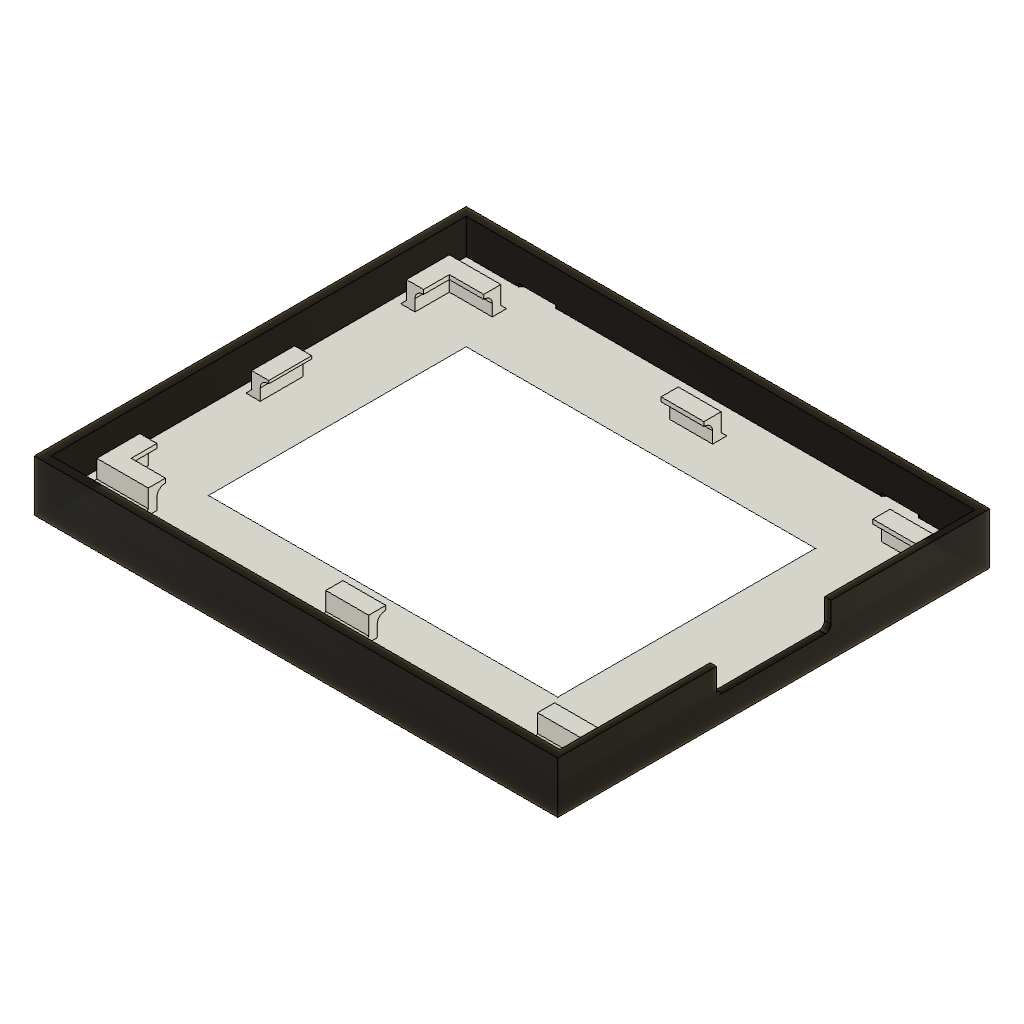
paperwhite_3 (Autodesk Fusion 360 design; units mm, degrees)
Autodesk Fusion 360 part; units mm, degrees
note: some values were not read from the file. Chosen so that the rebuilt part matches the saved one: which face or edge a step refers to; which pieces of a blend or face edit are solid. Set by a fixed rule: which sketch regions a step uses.
sketch "Sketch1" plane through (0, 0, 0) normal (0, 0, 1) x (1, 0, 0)
  line L0 (0, 0) -> (122, 0)
  line L1 (122, 0) -> (122, -90)
  line L2 (122, -90) -> (0, -90)
  line L3 (0, -90) -> (0, 0)
  line L4 (149.5, -117.5) -> (-27.5, -117.5)
  line L5 (-27.5, -117.5) -> (-27.5, 27.5)
  line L6 (-27.5, 27.5) -> (149.5, 27.5)
  line L7 (149.5, 27.5) -> (149.5, -117.5)
  line L8 (122, -45) -> (0, -45) construction
  line L9 (61, -45) -> (61, 0) construction
  line L10 (61, -45) -> (65, -45) construction
  line L11 (149.5, 13.6) -> (-19.5, 13.6)
  line L12 (-19.5, 13.6) -> (-19.5, -103.6)
  line L13 (-19.5, -103.6) -> (149.5, -103.6)
  line L14 (149.5, -103.6) -> (149.5, 13.6)
  line L15 (149.5, 13.6) -> (-19.5, -103.6) construction
  line L16 (-19.5, 13.6) -> (149.5, -103.6) construction
  line L17 (146.5, 13.6) -> (131.5, 13.6)
  line L18 (131.5, 13.6) -> (131.5, 16.6)
  line L19 (131.5, 16.6) -> (146.5, 16.6)
  line L20 (146.5, 16.6) -> (146.5, 13.6)
  line L21 (-24.5, 24.5) -> (146.5, 24.5)
  line L22 (146.5, 24.5) -> (146.5, -114.5)
  line L23 (146.5, -114.5) -> (-24.5, -114.5)
  line L24 (-24.5, -114.5) -> (-24.5, 24.5)
  line L25 (152.5, 30.5) -> (152.5, -120.5)
  line L26 (152.5, -120.5) -> (-30.5, -120.5)
  line L27 (-30.5, -120.5) -> (-30.5, 30.5)
  line L28 (-30.5, 30.5) -> (152.5, 30.5)
  line L29 (72.5, 13.6) -> (57.5, 13.6)
  line L30 (57.5, 13.6) -> (57.5, 16.6)
  line L31 (57.5, 16.6) -> (72.5, 16.6)
  line L32 (72.5, 16.6) -> (72.5, 13.6)
  line L33 (-19.5, 13.6) -> (-4.5, 13.6)
  line L34 (-4.5, 13.6) -> (-4.5, 16.6)
  line L35 (-4.5, 16.6) -> (-22.5, 16.6)
  line L36 (-19.5, -37.5) -> (-22.5, -37.5)
  line L37 (-22.5, -37.5) -> (-22.5, -52.5)
  line L38 (-22.5, -52.5) -> (-19.5, -52.5)
  line L39 (-19.5, -52.5) -> (-19.5, -37.5)
  line L40 (146.5, -103.6) -> (131.5, -103.6)
  line L41 (131.5, -103.6) -> (131.5, -106.6)
  line L42 (131.5, -106.6) -> (146.5, -106.6)
  line L43 (146.5, -106.6) -> (146.5, -103.6)
  line L44 (72.5, -103.6) -> (57.5, -103.6)
  line L45 (57.5, -103.6) -> (57.5, -106.6)
  line L46 (57.5, -106.6) -> (72.5, -106.6)
  line L47 (72.5, -106.6) -> (72.5, -103.6)
  line L48 (-4.5, -103.6) -> (-19.5, -103.6)
  line L49 (-19.5, -106.6) -> (-4.5, -106.6)
  line L50 (-4.5, -106.6) -> (-4.5, -103.6)
  line L51 (-19.5, -106.6) -> (-22.5, -106.6)
  line L52 (-22.5, -106.6) -> (-22.5, -91.6)
  line L53 (-22.5, -91.6) -> (-19.5, -91.6)
  line L54 (-19.5, -91.6) -> (-19.5, -103.6)
  line L55 (-22.5, 16.6) -> (-22.5, 1.6)
  line L56 (-22.5, 1.6) -> (-19.5, 1.6)
  line L57 (-19.5, 1.6) -> (-19.5, 13.6)
  line L58 (146.5, -103.6) -> (131.5, -103.6)
  line L59 (131.5, -103.6) -> (131.5, -100.6)
  line L60 (131.5, -100.6) -> (146.5, -100.6)
  line L61 (146.5, -100.6) -> (146.5, -103.6)
  line L62 (72.5, -103.6) -> (57.5, -103.6)
  line L63 (57.5, -103.6) -> (57.5, -100.6)
  line L64 (57.5, -100.6) -> (72.5, -100.6)
  line L65 (72.5, -100.6) -> (72.5, -103.6)
  line L66 (-4.5, -103.6) -> (-19.5, -103.6)
  line L67 (-16.5, -100.6) -> (-4.5, -100.6)
  line L68 (-4.5, -100.6) -> (-4.5, -103.6)
  line L69 (-19.5, -52.5) -> (-16.5, -52.5)
  line L70 (-16.5, -52.5) -> (-16.5, -37.5)
  line L71 (-16.5, -37.5) -> (-19.5, -37.5)
  line L72 (-19.5, -37.5) -> (-19.5, -52.5)
  line L73 (-19.5, -91.6) -> (-16.5, -91.6)
  line L74 (-16.5, -91.6) -> (-16.5, -100.6)
  line L75 (-4.5, 13.6) -> (-19.5, 13.6)
  line L76 (-16.5, 10.6) -> (-4.5, 10.6)
  line L77 (-4.5, 10.6) -> (-4.5, 13.6)
  line L78 (-19.5, 1.6) -> (-16.5, 1.6)
  line L79 (-19.5, 11) -> (-19.5, 1.6)
  line L80 (131.5, 16.6) -> (131.5, 10.6)
  line L81 (131.5, 10.6) -> (146.5, 10.6)
  line L82 (146.5, 10.6) -> (146.5, 13.6)
  line L83 (72.5, 13.6) -> (57.5, 13.6)
  line L84 (57.5, 13.6) -> (57.5, 10.6)
  line L85 (57.5, 10.6) -> (72.5, 10.6)
  line L86 (72.5, 10.6) -> (72.5, 13.6)
  line L87 (-16.5, 1.6) -> (-16.5, 10.6)
  point P0 (65, -45)
  dimension "d15" = 122
  dimension "d16" = 90
  dimension "d18" = 4
  dimension "d19" = 169
  dimension "d20" = 117.2
  dimension "d21" = 15
  dimension "d22" = 3
  dimension "d25" = 3
  dimension "d40" = 15
  dimension "d41" = 15
  dimension "d43" = 3
  dimension "d45" = 3
  dimension "d46" = 15
  dimension "d59" = 15
  dimension "d61" = 15
  dimension "d63" = 3
  dimension "d64" = 3
  dimension "d68" = 3
  dimension "d72" = 15
  dimension "d73" = 3
  dimension "d126" = 27.5
  dimension "d127" = 27.5
  dimension "d129" = 27.5
  dimension "d130" = 27.5
  constraint horizontal L0
  constraint vertical L1
  constraint horizontal L2
  constraint vertical L3
  constraint coincident L0.start L3.end
  constraint midpoint L1 L8.start
  constraint midpoint L3 L8.end
  constraint midpoint L8 L9.start
  constraint midpoint L0 L9.end
  constraint perpendicular L9 L10
  constraint horizontal L11
  constraint perpendicular L11 L12
  constraint parallel L11 L13
  constraint parallel L12 L14
  constraint coincident L15 P0
  constraint coincident L16 P0
  constraint coincident P0 L10.end
  constraint horizontal L17
  constraint vertical L18
  constraint horizontal L19
  constraint vertical L20
  constraint coincident L11 L17.start
  constraint horizontal L29
  constraint vertical L30
  constraint horizontal L31
  constraint vertical L32
  constraint coincident L11 L29.start
  constraint horizontal L33
  constraint vertical L34
  constraint horizontal L35
  constraint horizontal L36
  constraint vertical L37
  constraint horizontal L38
  constraint vertical L39
  constraint coincident L12 L36.start
  constraint horizontal L40
  constraint vertical L41
  constraint horizontal L42
  constraint vertical L43
  constraint coincident L13 L40.start
  constraint coincident L22 L40.start
  constraint horizontal L44
  constraint vertical L45
  constraint horizontal L46
  constraint vertical L47
  constraint coincident L13 L44.start
  constraint horizontal L48
  constraint horizontal L49
  constraint vertical L50
  constraint coincident L13 L48.start
  constraint horizontal L51
  constraint vertical L52
  constraint horizontal L53
  constraint vertical L54
  constraint vertical L55
  constraint horizontal L56
  constraint vertical L57
  constraint horizontal L58
  constraint vertical L59
  constraint horizontal L60
  constraint vertical L61
  constraint horizontal L62
  constraint vertical L63
  constraint horizontal L64
  constraint vertical L65
  constraint horizontal L66
  constraint horizontal L67
  constraint vertical L68
  constraint horizontal L69
  constraint vertical L70
  constraint horizontal L71
  constraint vertical L72
  constraint horizontal L73
  constraint vertical L74
  constraint horizontal L75
  constraint horizontal L76
  constraint vertical L77
  constraint horizontal L78
  constraint vertical L87
  constraint vertical L79
  constraint vertical L80
  constraint horizontal L81
  constraint vertical L82
  constraint horizontal L83
  constraint vertical L84
  constraint horizontal L85
  constraint vertical L86
  constraint coincident L20 L17.start
  constraint midpoint L13 L62
  constraint midpoint L11 L29
  constraint equal L53 L73
  constraint coincident L12 L13.start
  constraint midpoint L12 L72
  constraint equal L37 L70
  constraint equal L36 L71
  constraint equal L31 L85
  constraint equal L42 L60
  constraint equal L41 L59
  constraint equal L32 L86
  constraint equal L46 L64
  constraint equal L47 L65
  constraint equal L49 L52
  constraint equal L50 L68
  constraint equal L68 L73
  constraint equal L48 L52
  constraint equal L20 L82
  constraint equal L19 L81
  constraint coincident L19 L18.end
  constraint coincident L22 L17.start
  constraint equal L34 L77
  constraint coincident L11.end L12.start
  constraint equal L77 L78
  constraint equal L56 L78
  constraint equal L55 L75
  constraint coincident L11.end L12
  measures "d15" distance of L0.start L0.end
  measures "d16" distance of L0.start L2.end
  measures "d18" distance of L9.start P0
  measures "d19" distance of L12.end L13.end
  measures "d20" distance of L11.end L12.end
  measures "d21" distance of L17.start L17.end
  measures "d22" distance of L17.start L19.end
  measures "d40" distance of L11.end L33.end
  measures "d41" distance of L36.start L38.end
  measures "d43" distance of L40.start L42.end
  measures "d45" distance of L44.start L46.end
  measures "d46" distance of L48.start L12.end
  measures "d59" distance of L40.start L40.end
  measures "d61" distance of L44.start L44.end
  measures "d63" distance of L48.start L67.end
  measures "d64" distance of L38.end L69.end
  measures "d68" distance of L33.end L76.end
  measures "d72" distance of L29.start L29.end
  measures "d73" distance of L29.start L85.end
  measures "d126" distance of L0 L6
  measures "d127" distance of L2 L4
  measures "d129" distance of L1 L7
  measures "d130" distance of L3 L5
extrude "Extrude4" add sketch "Sketch1" along normal blind 1 contours L4 L5 L6 L7 L11 L13 L20 L21 L22 L23 L24 L43 | L7 L11 L13 L14 L22 L61 L82 | L13 L22 L40 L41 L42 L43 L58 | L13 L22 L40 L58 L59 L60 L61 | L11 L17 L22 L80 L81 L82 | L11 L17 L18 L19 L20 L22 L80 | L11 L12 L13 L18 L19 L21 L22 L23 L24 L30 L31 L32 L34 L35 L36 L37 L38 L41 L42 L45 L46 L47 L49 L50 L51 L52 L53 L55 L56 L80 | L11 L12 L13 L22 L59 L60 L63 L64 L65 L67 L68 L69 L70 L71 L73 L74 L76 L77 L78 L80 L81 L84 L85 L86 L87 | L13 L44 L45 L46 L47 L62 | L13 L44 L62 L63 L64 L65 | L11 L29 L83 L84 L85 L86 | L11 L29 L30 L31 L32 L83 | L12 L13 L48 L49 L50 L51 L52 L53 L54 L66 | L12 L13 L48 L54 L66 L67 L68 L73 L74 | L11 L12 L33 L57 L75 L76 L77 L78 L79 L87 | L11 L12 L33 L34 L35 L55 L56 L57 L75 L79 | L12 L36 L37 L38 L39 L72 | L12 L39 L69 L70 L71 L72 makes body 1
sketch "Sketch2" plane through (154.5, 0, 0) normal (1, 0, 0) x (0, 1, 0)
  line L0 (-122.5, 13) -> (-122.5, 0)
  line L1 (32.5, 0) -> (32.5, 13)
  line L2 (32.5, 13) -> (-122.5, 13)
  line L3 (27.5, 1) -> (-117.5, 1)
  line L4 (-45, 0) -> (-45, 13)
  line L5 (-45, 13) -> (-65, 13) construction
  line L6 (-65, 13) -> (-25, 13)
  line L7 (-25, 13) -> (-25, 3.8)
  line L8 (-25, 3.8) -> (-65, 3.8)
  line L9 (-65, 3.8) -> (-65, 13)
  line L10 (-122.5, 0) -> (32.5, 0)
  point P0 (-45, 0)
  dimension "d31" = 20
  dimension "d32" = 40
  dimension "d132" = 9.2
  constraint coincident P0 L4.start
  constraint perpendicular L3 L4
  constraint perpendicular L4 L5
  constraint horizontal L6
  constraint vertical L7
  constraint horizontal L8
  constraint vertical L9
  constraint coincident L2 L5.end
  measures "d31" distance of L4.end L5.end
  measures "d32" distance of L5.end L6.end
  measures "d132" distance of L6 L8
extrude "Extrude7" add sketch "Sketch1" against normal blind 5 separate body contours L4 L5 L6 L7 L11 L13 L20 L21 L22 L23 L24 L43 | L7 L11 L13 L14 L22 L61 L82 | L25 L26 L27 L28 makes body 2
extrude "Extrude8" add sketch "Sketch1" along normal blind 13 contours L25 L26 L27 L28 bodies 2
chamfer "Chamfer1" distance 1 angle 45 4 edges at (122, -45, 0) (61, 0, 0) (0, -45, 0) (61, -90, 0) on bodies 1
extrude "Extrude9" add sketch "Sketch1" along normal blind 7.8 from surface at 1 contours L13 L22 L40 L41 L42 L43 L58 | L11 L17 L18 L19 L20 L22 L80 | L13 L44 L45 L46 L47 L62 | L11 L29 L30 L31 L32 L83 | L12 L13 L48 L49 L50 L51 L52 L53 L54 L66 | L11 L12 L33 L34 L35 L55 L56 L57 L75 L79 | L12 L36 L37 L38 L39 L72 bodies 1
chamfer "Chamfer2" distance 2 angle 45 9 edges at (139, 16.6, 1) (65, 16.6, 1) (-13.5, 16.6, 1) (-22.5, 9.1, 1) (-22.5, -45, 1) (-22.5, -99.1, 1) (-13.5, -106.6, 1) (65, -106.6, 1) (139, -106.6, 1) on bodies 1
extrude "Extrude10" cut sketch "Sketch2" against normal blind 5 contours L2 L4 L6 L8 L9 | L2 L4 L6 L7 L8 bodies 2
fillet "Fillet1" radius 2 2 edges at (151, -65, 3.8) (151, -25, 3.8) on bodies 2
extrude "Extrude11" add sketch "Sketch1" against normal blind 1 from surface at 8.8 contours L13 L22 L40 L58 L59 L60 L61 | L11 L17 L22 L80 L81 L82 | L13 L44 L62 L63 L64 L65 | L11 L29 L83 L84 L85 L86 | L12 L13 L48 L54 L66 L67 L68 L73 L74 | L11 L12 L33 L57 L75 L76 L77 L78 L79 L87 | L12 L39 L69 L70 L71 L72 bodies 1
extrude "Extrude12" add 6 faces at (141.5, -104.6, 8.8) (62.5, -105.6, 8.8) (-20.5, -99.6, 8.8) (-14.5, 14.6, 8.8) (67.5, 13.6, 8.8) (141.5, 12.6, 8.8) along direction (0, 0, 1) blind 0.5 on bodies 1 bodies 1
move_face "OffsetFaces3" offset -0.2 4 faces at (31.5, 27.5, 0.6667) (149.5, -20.8333, 0.6667) (90.5, -117.5, 0.6667) (-27.5, -69.1667, 0.6667) on bodies 1
sketch "Sketch3" plane through (0, -117.5, 0) normal (0, 1, 0) x (-1, 0, 0)
  line L0 (-149.5, 0) -> (27.5, 0)
  line L1 (27.5, 0) -> (27.5, 13)
  line L2 (27.5, 13) -> (-149.5, 13)
  line L3 (-149.5, 13) -> (-149.5, 0)
  line L4 (-125, 1) -> (-62, 1)
  line L5 (-62, 1) -> (-62, -9)
  line L6 (-62, -9) -> (-125, -9)
  line L7 (-125, -9) -> (-125, 1)
  line L8 (27.3, 1) -> (-149.3, 1)
  line L9 (-125, 1) -> (-115, 1)
  line L10 (-115, 1) -> (-115, 3)
  line L11 (-115, 3) -> (-125, 3)
  line L12 (-125, 3) -> (-125, 1)
  dimension "d80" = 10
  dimension "d81" = 2
  constraint horizontal L4
  constraint vertical L5
  constraint horizontal L6
  constraint vertical L7
  constraint coincident L4.start L8
  constraint horizontal L9
  constraint vertical L10
  constraint horizontal L11
  constraint vertical L12
  measures "d80" distance of L4.start L9.end
  measures "d81" distance of L4.start L11.end
fillet "Fillet2" radius 2.75 9 edges at (65, 13.6, 7.8) (139, 13.6, 7.8) (-12, 13.6, 7.8) (-19.5, 7.6, 7.8) (-19.5, -45, 7.8) (-12, -103.6, 7.8) (-19.5, -97.6, 7.8) (65, -103.6, 7.8) (139, -103.6, 7.8) on bodies 1
sketch "Sketch4" plane through (0, 0, 1) normal (0, 0, 1) x (-1, 0, 0)
  line L0 (-149.3, 117.3) -> (-149.3, -27.3)
  line L1 (-149.3, -27.3) -> (27.3, -27.3)
  line L2 (27.3, 117.3) -> (-149.3, 117.3)
  line L3 (-122, 0) -> (-122, 90)
  line L4 (27.5, 45) -> (-149.3, 45) construction
  line L5 (7.5, -27.3) -> (-2.5, -27.3)
  line L6 (-2.5, -27.3) -> (-2.5, -28.8)
  line L7 (-2.5, -28.8) -> (7.5, -28.8)
  line L8 (7.5, -28.8) -> (7.5, -27.3)
  line L9 (-129.3, -27.3) -> (-119.3, -27.3)
  line L10 (-119.3, -27.3) -> (-119.3, -28.8)
  line L11 (-119.3, -28.8) -> (-129.3, -28.8)
  line L12 (-129.3, -28.8) -> (-129.3, -27.3)
  line L13 (7.5, -28.8) -> (9, -27.3)
  line L14 (7.5, -28.8) -> (9.6213, -28.8) construction
  line L15 (-2.5, -28.8) -> (-4, -27.3)
  line L16 (-119.3, -28.8) -> (-117.8, -27.3)
  line L17 (-129.3, -28.8) -> (-130.8, -27.3)
  line L18 (7.5, 118.8) -> (7.5, 117.3)
  line L19 (7.5, 118.8) -> (9, 117.3)
  line L20 (-2.5, 118.8) -> (7.5, 118.8)
  line L21 (7.5, 117.3) -> (-2.5, 117.3)
  line L22 (-2.5, 117.3) -> (-2.5, 118.8)
  line L23 (-2.5, 118.8) -> (-4, 117.3)
  line L24 (-119.3, 118.8) -> (-117.8, 117.3)
  line L25 (-119.3, 117.3) -> (-119.3, 118.8)
  line L26 (-129.3, 117.3) -> (-119.3, 117.3)
  line L27 (-119.3, 118.8) -> (-129.3, 118.8)
  line L28 (-129.3, 118.8) -> (-129.3, 117.3)
  line L29 (-129.3, 118.8) -> (-130.8, 117.3)
  line L30 (27.5, 117.5) -> (27.5, -27.5)
  line L31 (-131.5, 108.6) -> (-131.5, 103.6)
  line L32 (-131.5, 103.6) -> (-146.5, 103.6)
  line L33 (-146.5, 103.6) -> (-146.5, 108.6)
  line L34 (-146.5, 108.6) -> (-131.5, 108.6)
  line L35 (-146.5, -18.6) -> (-146.5, -13.6)
  line L36 (-146.5, -13.6) -> (-131.5, -13.6)
  line L37 (-131.5, -13.6) -> (-131.5, -18.6)
  line L38 (-131.5, -18.6) -> (-146.5, -18.6)
  line L39 (-57.5, 108.6) -> (-57.5, 103.6)
  line L40 (-57.5, 103.6) -> (-72.5, 103.6)
  line L41 (-72.5, 103.6) -> (-72.5, 108.6)
  line L42 (-72.5, 108.6) -> (-57.5, 108.6)
  line L43 (-72.5, -18.6) -> (-72.5, -13.6)
  line L44 (-72.5, -13.6) -> (-57.5, -13.6)
  line L45 (-57.5, -13.6) -> (-57.5, -18.6)
  line L46 (-57.5, -18.6) -> (-72.5, -18.6)
  line L47 (27.3, -27.3) -> (27.3, 117.3)
  line L48 (-122, 90) -> (0, 90)
  line L49 (0, 90) -> (0, 0)
  line L50 (0, 0) -> (-122, 0)
  line L51 (4.5, 103.6) -> (4.5, 108.6)
  line L52 (4.5, 108.6) -> (24.5, 108.6)
  line L53 (24.5, 91.6) -> (19.5, 91.6)
  line L54 (19.5, 91.6) -> (19.5, 103.6)
  line L55 (19.5, 103.6) -> (4.5, 103.6)
  line L56 (19.5, -1.6) -> (24.5, -1.6)
  line L57 (24.5, -18.6) -> (4.5, -18.6)
  line L58 (4.5, -18.6) -> (4.5, -13.6)
  line L59 (4.5, -13.6) -> (19.5, -13.6)
  line L60 (19.5, -13.6) -> (19.5, -1.6)
  line L61 (24.5, 37.5) -> (19.5, 37.5)
  line L62 (19.5, 37.5) -> (19.5, 52.5)
  line L63 (19.5, 52.5) -> (24.5, 52.5)
  line L64 (24.5, 108.6) -> (24.5, 91.6)
  line L65 (24.5, -1.6) -> (24.5, -18.6)
  line L66 (24.5, 52.5) -> (24.5, 37.5)
  dimension "d84" = 10
  dimension "d85" = 1.5
  dimension "d86" = 10
  dimension "d87" = 1.5
  dimension "d88" = 45
  dimension "d121" = 20
  dimension "d122" = 20
  constraint midpoint L0 L4.end
  constraint horizontal L5
  constraint vertical L6
  constraint horizontal L7
  constraint vertical L8
  constraint coincident L1 L5.start
  constraint horizontal L9
  constraint vertical L10
  constraint horizontal L11
  constraint vertical L12
  constraint coincident L1 L9.start
  constraint horizontal L14
  constraint coincident L1 L13.end
  constraint coincident L1 L15.end
  constraint perpendicular L13 L15
  constraint coincident L1 L16.end
  constraint perpendicular L15 L16
  constraint coincident L1 L17.end
  constraint perpendicular L16 L17
  constraint symmetric L4 L5.start L18.end
  constraint symmetric L4 L5.end L21.end
  constraint symmetric L4 L6.end L20.start
  constraint symmetric L4 L7.end L18.start
  constraint symmetric L4 L9.start L26.start
  constraint symmetric L4 L9.end L25.start
  constraint symmetric L4 L10.end L24.start
  constraint symmetric L4 L11.end L27.end
  constraint symmetric L4 L13.end L19.end
  constraint symmetric L4 L15.end L23.end
  constraint symmetric L4 L16.end L24.end
  constraint symmetric L4 L17.end L29.end
  constraint midpoint L4.start L30
  measures "d84" distance of L5.start L5.end
  measures "d85" distance of L5.start L7.end
  measures "d86" distance of L9.start L9.end
  measures "d87" distance of L9.start L11.end
  measures "d88" angle of L13 L14
  measures "d121" distance of L8 L30
  measures "d122" distance of L0 L12
extrude "Extrude13" add 1 faces at (149.3, -20.9, 0.6667) along direction (1, 0, 0) blind 0.75 on bodies 1 bodies 1
extrude "Extrude14" cut 1 faces at (149.5, 10, 6.2667) along direction (1, 0, 0) blind 0.75 on bodies 2 bodies 2
extrude "Extrude15" add sketch "Sketch4" against normal blind 1 contours L2 L28 L29 | L1 L12 L17 | L2 L25 L26 L27 L28 | L1 L9 L10 L11 L12 | L2 L24 L25 | L1 L10 L16 | L2 L22 L23 | L1 L6 L15 | L2 L18 L20 L21 L22 | L1 L5 L6 L7 L8 | L2 L18 L19 | L1 L8 L13 bodies 1
chamfer "Chamfer3" distance 0.3 angle 45 8 edges at (124.3, 28.8, 1) (124.3, 28.8, 0) (-2.5, 28.8, 1) (-2.5, 28.8, 0) (124.3, -118.8, 1) (124.3, -118.8, 0) (-2.5, -118.8, 1) (-2.5, -118.8, 0) on bodies 1
combine "Combine2" operation cut target body 2 tool bodies 1 keep tools
move_face "OffsetFaces4" offset -0.3 24 faces at (126.0667, -117.8333, 1) (130.2667, -117.8333, 0.6667) (125.9667, -118.6, 0.9) (122.6333, -118.8, 0.5667) (125.9667, -118.6, 0.1) (118.3333, -117.8333, 0.3333) (126.0667, 27.8333, 1) (130.2667, 27.8333, 0.3333) (125.9667, 28.6, 0.9) (122.6333, 28.8, 0.5667) (125.9667, 28.6, 0.1) (118.6667, 28.1667, 0.6667) (-8.4667, 27.8333, 0.3333) (-0.8333, 28.6, 0.1) (-0.8333, 28.8, 0.4333) (3.1333, 28.1667, 0.3333) (-0.7333, 27.8333, 1) (-0.8333, 28.6, 0.9) (-0.7333, -117.8333, 1) (-0.8333, -118.6, 0.9) (-8.4667, -117.8333, 0.3333) (3.4667, -117.8333, 0.6667) (-0.8333, -118.8, 0.5667) (-0.8333, -118.6, 0.1) on bodies 2
chamfer "Chamfer4" distance 0.5 angle 45 4 edges at (-2.5, -117.5, 1.3) (124.3, -117.5, 1.3) (124.3, 27.5, 1.3) (-2.5, 27.5, 1.3) on bodies 2
chamfer "Chamfer5" distance 3 distance2 5 4 edges at (146.5, -45, -5) (61, 24.5, -5) (61, -114.5, -5) (-24.5, -45, -5) measured on face at (89.5, -118.5, -5) measured on face at (89.5, -118.5, -5) measured on face at (89.5, -118.5, -5) measured on face at (89.5, -118.5, -5) on bodies 2
equation "d15 = screen_height"
equation "d16 = screen_width"
equation "d18 = ( screen_bott_padding - screen_top_padding ) / 2"
equation "d19 = kindle_height"
equation "d20 = kindle_width"
equation "d21 = holder_lengh"
equation "d22 = holder_width"
equation "d25 = bezel_width"
equation "d26 = -( bezel_width )"
equation "d40 = holder_lengh"
equation "d41 = holder_lengh"
equation "d43 = holder_width"
equation "d45 = holder_width"
equation "d46 = holder_lengh"
equation "d59 = holder_lengh"
equation "d61 = holder_lengh"
equation "d63 = holder_width"
equation "d64 = holder_width"
equation "d68 = holder_width"
equation "d72 = holder_lengh"
equation "d73 = holder_width"
equation "bezel_width = 3 mm" comment "3.00"
equation "screen_width = 90 mm" comment "90.00"
equation "screen_height = 122 mm" comment "122.00"
equation "kindle_height = 169 mm" comment "169.00"
equation "kindle_width = 117.2 mm" comment "117.20"
equation "screen_bott_padding = 27.5 mm" comment "27.50"
equation "screen_top_padding = 19.5 mm" comment "19.50"
equation "holder_lengh = 15 mm" comment "15.00"
equation "holder_width = 3 mm" comment "3.00"
equation "screen_side_padding = ( kindle_width - screen_width ) / 2" comment "13.60"
equation "carton_bezel_padding_horizontal = 13.9 mm" comment "13.90"
equation "d126 = screen_side_padding + carton_bezel_padding_horizontal"
equation "d127 = screen_side_padding + carton_bezel_padding_horizontal"
equation "carton_bezel_padding_vertical = screen_bott_padding" comment "27.50"
equation "d129 = carton_bezel_padding_vertical"
equation "d130 = carton_bezel_padding_vertical"
